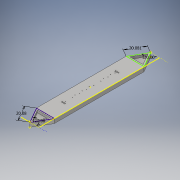
# Autodesk Inventor part: top
Saved by Autodesk Inventor 2016 (Build 200138000, 138)
## iProperties
Created: 2015-12-05
Part Number: top
Material: Generic
Document SubType Name: Modeling
Designer: acd
Density: 1 g/cm^3
Appearance: Default
Surface Area: 7060.29 cm^2
Author: acd
Autodesk Inventor part; units mm, degrees
sketch "Sketch1" plane through (0, 0, 0) normal (0, 1, 0) x (-1, 0, 0)
  line L0 (-100.4, 678.442) -> (100.4, 678.442)
  line L1 (100.4, 678.442) -> (100.4, -678.442)
  line L2 (100.4, -678.442) -> (-100.4, -678.442)
  line L3 (-100.4, -678.442) -> (-100.4, 678.442)
  line L4 (-100.4, 678.442) -> (100.4, -678.442) construction
  line L5 (100.4, 678.442) -> (-100.4, -678.442) construction
  point P0 (0, 0)
  dimension "d0" = 200.8
  dimension "d1" = 1356.884
  constraints: 12 end point, 2 midpoint, 2 parallel, 1 horizontal, 1 perpendicular
  measures "d0" distance of L1.end L2.end
  measures "d1" distance of L0.end L1.end
extrude "Extrusion1" add sketch "Sketch1" along normal blind 50.8
sketch "Sketch2" plane through (0, 50.8, 0) normal (0, 1, 0) x (1, 0, 0)
  line L0 (-100.4, -678.442) -> (100.4, -678.442) projected
  line L1 (0, -678.442) -> (-100.4, -504.5441)
  line L2 (0, -678.442) -> (200.8, -678.442) construction
  line L3 (-100.4, -504.5441) -> (100.4, -504.5441)
  line L4 (100.4, -678.442) -> (100.4, 678.442) projected
  line L5 (0, -678.442) -> (100.4, -504.5441)
  line L6 (0, 678.442) -> (-100.4062, 504.5334)
  line L7 (0, 678.442) -> (200.8124, 678.442) construction
  line L8 (-100.4062, 504.5334) -> (100.4, 504.5334)
  line L9 (0, 678.442) -> (100.4, 504.5334)
  point P0 (0, 0)
  dimension "d10" = 150
  dimension "d11" = 150
  dimension "d12" = 60
  dimension "d4" = 200.8
  dimension "d5" = 120
  dimension "d6" = 200.8124
  dimension "d7" = 120
  constraints: 16 end point, 3 horizontal, 2 equal length, 2 point on line, 1 midpoint, 1 perpendicular
  measures "d4" distance of L1.start L1.end
  measures "d5" angle of L2 L1
  measures "d6" distance of L6.start L6.end
  measures "d7" angle of L6 L7
ref_plane "Work Plane1" through (0, 50.8, 678.442) normal (0.866, 0, 0.5) x (0, -1, 0)
split "Split1" plane through (0, 50.8, 678.442) removes the side toward (0.866, 0, 0.5)
ref_plane "Work Plane2" through (0, 0, 678.442) normal (-0.866, 0, 0.5) x (0, 1, 0)
ref_plane "Work Plane3" through (0, 0, -678.442) normal (0.866, 0, 0.5) x (0, 1, 0)
split "Split2" plane through (0, 0, -678.442) removes the side toward (-0.866, 0, -0.5)
split "Split3" plane through (0, 0, 678.442) removes the side toward (-0.866, 0, 0.5)
ref_plane "Work Plane4" through (0, 0, -678.442) normal (0.866, 0, -0.5) x (0, 1, 0)
split "Split4" plane through (0, 0, -678.442) removes the side toward (0.866, 0, -0.5)
sketch "Sketch3" plane through (0, 50.8, 0) normal (0, 1, 0) x (1, 0, 0)
  line L0 (-75, -519.2088) -> (75, -519.2088)
  line L1 (75, -519.2088) -> (0, -649.1126)
  line L2 (0, -649.1126) -> (-75, -519.2088)
  line L3 (-75.0016, 519.2007) -> (74.9984, 519.2007)
  line L4 (74.9984, 519.2007) -> (-0.0016, 649.1046)
  line L5 (-0.0016, 649.1046) -> (-75.0016, 519.2007)
  circle A0 centre (-0.0016, 562.502) radius 43.3013
  circle A1 centre (-0.0016, 562.502) radius 57.9687
  point P0 (0, 0)
  dimension "d6" = 200.8124
  dimension "d7" = 120
  dimension "d8" = 150
  dimension "d9" = 150
  dimension "d10" = 150
  dimension "d11" = 150
  dimension "d12" = 60
  constraints: 12 end point, 3 tangent, 2 centre point, 1 coincident, 1 horizontal, 3 other
  measures "d8" distance of L0.start L0.end
  measures "d9" distance of L0.end L1.end
  measures "d10" distance of L3.start L3.end
  measures "d11" distance of L3.end L4.end
  measures "d12" angle of L4 L3
sketch "Sketch4" plane through (0, 50.8, 0) normal (0, 1, 0) x (1, 0, 0)
  point P0 (0, 0)
sketch "Sketch5" plane through (0, 50.8, 0) normal (0, 1, 0) x (1, 0, 0)
  point P0 (0, 0)
extrude "Extrusion2" cut sketch "Sketch3" against normal blind 25.4 contours L0 L1 L2
sketch "Sketch6" plane through (0, 50.8, 0) normal (0, 1, 0) x (1, 0, 0)
  line L0 (-75.0016, 519.2007) -> (74.9984, 519.2007)
  line L1 (74.9984, 519.2007) -> (-0.0016, 649.1046)
  line L2 (-0.0016, 649.1046) -> (-75.0016, 519.2007)
  point P0 (0, 0)
  dimension "d15" = 150
  dimension "d16" = 150
  constraints: 6 end point, 1 horizontal
  measures "d15" distance of L0.start L0.end
  measures "d16" distance of L0.end L1.end
extrude "Extrusion3" cut sketch "Sketch6" against normal blind 25.4
sketch "Sketch11" plane through (0, 50.8, 0) normal (0, 1, 0) x (1, 0, 0)
  line L0 (-20, 295) -> (20, 295)
  line L1 (20, 295) -> (20, 305)
  line L2 (20, 305) -> (-20, 305)
  line L3 (-20, 305) -> (-20, 295)
  line L4 (-20, 295) -> (20, 305) construction
  line L5 (20, 295) -> (-20, 305) construction
  point P0 (0, 0)
  point P1 (0, 300)
  dimension "d42" = 40
  dimension "d43" = 10
  constraints: 12 end point, 2 midpoint, 2 parallel, 1 horizontal, 1 perpendicular
  measures "d42" distance of L2.end L1.end
  measures "d43" distance of L1.end L0.end
extrude "Extrusion6" cut sketch "Sketch11" against normal blind 50.8
sketch "Sketch12" plane through (0, 50.8, 0) normal (0, 1, 0) x (1, 0, 0)
  line L0 (-20, -305) -> (20, -305)
  line L1 (20, -305) -> (20, -295)
  line L2 (20, -295) -> (-20, -295)
  line L3 (-20, -295) -> (-20, -305)
  line L4 (-20, -305) -> (20, -295) construction
  line L5 (20, -305) -> (-20, -295) construction
  point P0 (0, 0)
  point P1 (0, -300)
  dimension "d46" = 40
  dimension "d47" = 10
  constraints: 12 end point, 2 midpoint, 2 parallel, 1 horizontal, 1 perpendicular
  measures "d46" distance of L2.end L1.end
  measures "d47" distance of L1.end L0.end
extrude "Extrusion7" cut sketch "Sketch12" against normal blind 50.8
sketch "Sketch13" plane through (0, 50.8, 0) normal (0, 1, 0) x (1, 0, 0)
  circle A0 centre (0, -40) radius 2.5
  circle A1 centre (0, -120) radius 2.5
  circle A2 centre (0, -200) radius 2.5
  circle A3 centre (0, -280) radius 2.5
  circle A4 centre (0, 40) radius 2.5
  circle A5 centre (0, 100) radius 2.5
  circle A6 centre (0, 200) radius 2.5
  point P0 (0, 0)
  dimension "d50" = 5
  dimension "d51" = 5
  dimension "d52" = 5
  dimension "d53" = 5
  dimension "d54" = 5
  dimension "d55" = 5
  dimension "d56" = 5
  constraints: 7 centre point
  measures "d50" diameter of A0
  measures "d51" diameter of A1
  measures "d52" diameter of A2
  measures "d53" diameter of A3
  measures "d54" diameter of A4
  measures "d55" diameter of A5
  measures "d56" diameter of A6
extrude "Extrusion8" cut sketch "Sketch13" against normal blind 50.8 contours A3
sketch "Sketch14" plane through (0, 50.8, 0) normal (0, 1, 0) x (1, 0, 0)
  circle A0 centre (0, -200) radius 2.5
  point P0 (0, 0)
  dimension "d59" = 5
  constraints: 1 centre point
  measures "d59" diameter of A0
extrude "Extrusion9" cut sketch "Sketch14" against normal blind 50.8
sketch "Sketch15" plane through (0, 50.8, 0) normal (0, 1, 0) x (1, 0, 0)
  circle A0 centre (0, -120) radius 2.5
  point P0 (0, 0)
  dimension "d62" = 5
  constraints: 1 centre point
  measures "d62" diameter of A0
extrude "Extrusion10" cut sketch "Sketch15" against normal blind 50.8
sketch "Sketch16" plane through (0, 50.8, 0) normal (0, 1, 0) x (1, 0, 0)
  circle A0 centre (0, -40) radius 2.5
  circle A1 centre (0, 40) radius 2.5
  point P0 (0, 0)
  dimension "d65" = 5
  dimension "d66" = 5
  constraints: 2 centre point
  measures "d65" diameter of A0
  measures "d66" diameter of A1
extrude "Extrusion11" cut sketch "Sketch16" against normal blind 50.8
sketch "Sketch17" plane through (0, 50.8, 0) normal (0, 1, 0) x (1, 0, 0)
  circle A0 centre (0, 120) radius 2.5
  circle A1 centre (0, 200) radius 2.5
  circle A2 centre (0, 280) radius 2.5
  point P0 (0, 0)
  dimension "d69" = 5
  dimension "d70" = 5
  dimension "d71" = 5
  constraints: 3 centre point
  measures "d69" diameter of A0
  measures "d70" diameter of A1
  measures "d71" diameter of A2
extrude "Extrusion12" cut sketch "Sketch17" against normal blind 50.8
sketch "Sketch18" plane through (0, 0, 0) normal (0, -1, 0) x (1, 0, 0)
  circle A0 centre (-10, -240) radius 2.5
  circle A1 centre (-10, -160) radius 2.5
  circle A2 centre (-10, 0) radius 2.5
  circle A3 centre (-10, 80) radius 2.5
  circle A4 centre (-10, 160) radius 2.5
  point P0 (0, 0)
  dimension "d74" = 5
  dimension "d75" = 5
  dimension "d76" = 5
  dimension "d77" = 5
  dimension "d78" = 5
  constraints: 5 centre point
  measures "d74" diameter of A0
  measures "d75" diameter of A1
  measures "d76" diameter of A2
  measures "d77" diameter of A3
  measures "d78" diameter of A4
extrude "Extrusion13" cut sketch "Sketch18" against normal blind 50.8
sketch "Sketch19" plane through (0, 0, 0) normal (0, -1, 0) x (1, 0, 0)
  line L0 (74.9984, -519.2007) -> (-75.0016, -519.2007) projected
  line L1 (75.0016, 519.2007) -> (-75.0016, 519.2007)
  line L2 (-75.0016, 519.2007) -> (-75.0016, -519.2007)
  line L3 (-75.0016, -519.2007) -> (75.0016, -519.2007)
  line L4 (75.0016, -519.2007) -> (75.0016, 519.2007)
  line L5 (75.0016, 519.2007) -> (-75.0016, -519.2007) construction
  line L6 (-75.0016, 519.2007) -> (75.0016, -519.2007) construction
  point P0 (0, 0)
  constraints: 12 end point, 2 midpoint, 2 parallel, 1 horizontal, 1 perpendicular
extrude "Extrusion14" cut sketch "Sketch19" against normal blind 25.4
body "Solid1"
